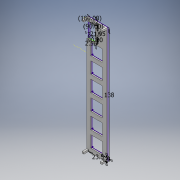
# Autodesk Inventor part: case-top
Saved by Autodesk Inventor 2017 (Build 210142000, 142)
## iProperties
Created: 2026-06-28
Part Number: case-top
Material: Generic
Document SubType Name: Modeling
Designer: hashire umamusume
Density: 1 g/cm^3
Appearance: Default
Author: hashire umamusume
Autodesk Inventor part; units mm, degrees
ref_plane "YZ Plane" through (0, 0, 0) normal (1, 0, 0) x (0, 1, 0)
ref_plane "XZ Plane" through (0, 0, 0) normal (0, 1, 0) x (-1, 0, 0)
ref_plane "XY Plane" through (0, 0, 0) normal (0, 0, 1) x (1, 0, 0)
sketch "keys" plane through (0, 0, 0) normal (0, 0, 1) x (1, 0, 0)
  line L0 (3.025, -2.525) -> (16.025, -2.525)
  line L1 (3.025, -16.525) -> (16.025, -16.525)
  line L2 (2.525, -3.025) -> (2.525, -16.025)
  line L3 (16.525, -3.025) -> (16.525, -16.025)
  arc A0 (3.025, -2.525) -> (2.525, -3.025) centre (3.025, -3.025) ccw
  arc A1 (16.525, -3.025) -> (16.025, -2.525) centre (16.025, -3.025) ccw
  arc A2 (2.525, -16.025) -> (3.025, -16.525) centre (3.025, -16.025) ccw
  arc A3 (16.025, -16.525) -> (16.525, -16.025) centre (16.025, -16.025) ccw
  line L4 (22.075, -2.525) -> (35.075, -2.525)
  line L5 (22.075, -16.525) -> (35.075, -16.525)
  line L6 (21.575, -3.025) -> (21.575, -16.025)
  line L7 (35.575, -3.025) -> (35.575, -16.025)
  arc A4 (22.075, -2.525) -> (21.575, -3.025) centre (22.075, -3.025) ccw
  arc A5 (35.575, -3.025) -> (35.075, -2.525) centre (35.075, -3.025) ccw
  arc A6 (21.575, -16.025) -> (22.075, -16.525) centre (22.075, -16.025) ccw
  arc A7 (35.075, -16.525) -> (35.575, -16.025) centre (35.075, -16.025) ccw
  line L8 (41.125, -2.525) -> (54.125, -2.525)
  line L9 (41.125, -16.525) -> (54.125, -16.525)
  line L10 (40.625, -3.025) -> (40.625, -16.025)
  line L11 (54.625, -3.025) -> (54.625, -16.025)
  arc A8 (41.125, -2.525) -> (40.625, -3.025) centre (41.125, -3.025) ccw
  arc A9 (54.625, -3.025) -> (54.125, -2.525) centre (54.125, -3.025) ccw
  arc A10 (40.625, -16.025) -> (41.125, -16.525) centre (41.125, -16.025) ccw
  arc A11 (54.125, -16.525) -> (54.625, -16.025) centre (54.125, -16.025) ccw
  line L12 (60.175, -2.525) -> (73.175, -2.525)
  line L13 (60.175, -16.525) -> (73.175, -16.525)
  line L14 (59.675, -3.025) -> (59.675, -16.025)
  line L15 (73.675, -3.025) -> (73.675, -16.025)
  arc A12 (60.175, -2.525) -> (59.675, -3.025) centre (60.175, -3.025) ccw
  arc A13 (73.675, -3.025) -> (73.175, -2.525) centre (73.175, -3.025) ccw
  arc A14 (59.675, -16.025) -> (60.175, -16.525) centre (60.175, -16.025) ccw
  arc A15 (73.175, -16.525) -> (73.675, -16.025) centre (73.175, -16.025) ccw
  line L16 (79.225, -2.525) -> (92.225, -2.525)
  line L17 (79.225, -16.525) -> (92.225, -16.525)
  line L18 (78.725, -3.025) -> (78.725, -16.025)
  line L19 (92.725, -3.025) -> (92.725, -16.025)
  arc A16 (79.225, -2.525) -> (78.725, -3.025) centre (79.225, -3.025) ccw
  arc A17 (92.725, -3.025) -> (92.225, -2.525) centre (92.225, -3.025) ccw
  arc A18 (78.725, -16.025) -> (79.225, -16.525) centre (79.225, -16.025) ccw
  arc A19 (92.225, -16.525) -> (92.725, -16.025) centre (92.225, -16.025) ccw
  line L20 (98.275, -2.525) -> (111.275, -2.525)
  line L21 (98.275, -16.525) -> (111.275, -16.525)
  line L22 (97.775, -3.025) -> (97.775, -16.025)
  line L23 (111.775, -3.025) -> (111.775, -16.025)
  arc A20 (98.275, -2.525) -> (97.775, -3.025) centre (98.275, -3.025) ccw
  arc A21 (111.775, -3.025) -> (111.275, -2.525) centre (111.275, -3.025) ccw
  arc A22 (97.775, -16.025) -> (98.275, -16.525) centre (98.275, -16.025) ccw
  arc A23 (111.275, -16.525) -> (111.775, -16.025) centre (111.275, -16.025) ccw
  point P0 (57.15, -9.525)
sketch "Sketch1" plane through (0, 0, 0) normal (0, 1, 0) x (-1, 0, 0)
  line L0 (0, 0) -> (-23.5, 0)
  line L1 (-23.5, 0) -> (-23.5, -138)
  line L2 (-23.5, -138) -> (0, -138)
  line L3 (0, -138) -> (0, 0)
  line L4 (-2, -2) -> (-21.5, -2)
  line L5 (-21.5, -2) -> (-21.5, -136)
  line L6 (-21.5, -136) -> (-2, -136)
  line L7 (-2, -136) -> (-2, -2)
  line L8 (-2, -2) -> (0, -2)
  line L9 (0, -2) -> (0, 0)
  line L10 (0, 0) -> (-2, 0)
  line L11 (-2, 0) -> (-2, -2)
  line L12 (-21.5, -2) -> (-23.5, -2)
  line L13 (-23.5, -2) -> (-23.5, 0)
  line L14 (-23.5, 0) -> (-21.5, 0)
  line L15 (-21.5, 0) -> (-21.5, -2)
  line L16 (-21.5, -136) -> (-23.5, -136)
  line L17 (-23.5, -136) -> (-23.5, -138)
  line L18 (-23.5, -138) -> (-21.5, -138)
  line L19 (-21.5, -138) -> (-21.5, -136)
  line L20 (-2, -136) -> (0, -136)
  line L21 (0, -136) -> (0, -138)
  line L22 (0, -138) -> (-2, -138)
  line L23 (-2, -138) -> (-2, -136)
  line L24 (-2, -38.4581) -> (17.5, -38.4581) construction
  line L25 (-21.5, -23.95) -> (-2, -23.95)
  line L26 (-2, -4.3088) -> (-10, -4.3088)
  line L27 (-2, -4.3088) -> (6, -4.3088) construction
  line L28 (-10, -4.3088) -> (-10, -22.3088)
  line L29 (-10, -22.3088) -> (-2, -22.3088)
  line L30 (-2, -4.3088) -> (0, -4.3088)
  line L31 (0, -4.3088) -> (0, -22.3088)
  line L32 (0, -22.3088) -> (-2, -22.3088)
  line L33 (-2, -22.3088) -> (-2, -4.3088)
  line L34 (0, -19.05) -> (0, 0)
  line L35 (-18.55, -132.7) -> (-18.55, -119.7)
  line L36 (-4.55, -132.7) -> (-4.55, -119.7)
  line L37 (-18.05, -133.2) -> (-5.05, -133.2)
  line L38 (-18.05, -119.2) -> (-5.05, -119.2)
  arc A0 (-18.55, -132.7) -> (-18.05, -133.2) centre (-18.05, -132.7) ccw
  arc A1 (-18.05, -119.2) -> (-18.55, -119.7) centre (-18.05, -119.7) ccw
  arc A2 (-5.05, -133.2) -> (-4.55, -132.7) centre (-5.05, -132.7) ccw
  arc A3 (-4.55, -119.7) -> (-5.05, -119.2) centre (-5.05, -119.7) ccw
  line L39 (-18.55, -113.65) -> (-18.55, -100.65)
  line L40 (-4.55, -113.65) -> (-4.55, -100.65)
  line L41 (-18.05, -114.15) -> (-5.05, -114.15)
  line L42 (-18.05, -100.15) -> (-5.05, -100.15)
  arc A4 (-18.55, -113.65) -> (-18.05, -114.15) centre (-18.05, -113.65) ccw
  arc A5 (-18.05, -100.15) -> (-18.55, -100.65) centre (-18.05, -100.65) ccw
  arc A6 (-5.05, -114.15) -> (-4.55, -113.65) centre (-5.05, -113.65) ccw
  arc A7 (-4.55, -100.65) -> (-5.05, -100.15) centre (-5.05, -100.65) ccw
  line L43 (-18.55, -94.6) -> (-18.55, -81.6)
  line L44 (-4.55, -94.6) -> (-4.55, -81.6)
  line L45 (-18.05, -95.1) -> (-5.05, -95.1)
  line L46 (-18.05, -81.1) -> (-5.05, -81.1)
  arc A8 (-18.55, -94.6) -> (-18.05, -95.1) centre (-18.05, -94.6) ccw
  arc A9 (-18.05, -81.1) -> (-18.55, -81.6) centre (-18.05, -81.6) ccw
  arc A10 (-5.05, -95.1) -> (-4.55, -94.6) centre (-5.05, -94.6) ccw
  arc A11 (-4.55, -81.6) -> (-5.05, -81.1) centre (-5.05, -81.6) ccw
  line L47 (-18.55, -75.55) -> (-18.55, -62.55)
  line L48 (-4.55, -75.55) -> (-4.55, -62.55)
  line L49 (-18.05, -76.05) -> (-5.05, -76.05)
  line L50 (-18.05, -62.05) -> (-5.05, -62.05)
  arc A12 (-18.55, -75.55) -> (-18.05, -76.05) centre (-18.05, -75.55) ccw
  arc A13 (-18.05, -62.05) -> (-18.55, -62.55) centre (-18.05, -62.55) ccw
  arc A14 (-5.05, -76.05) -> (-4.55, -75.55) centre (-5.05, -75.55) ccw
  arc A15 (-4.55, -62.55) -> (-5.05, -62.05) centre (-5.05, -62.55) ccw
  line L51 (-18.55, -56.5) -> (-18.55, -43.5)
  line L52 (-4.55, -56.5) -> (-4.55, -43.5)
  line L53 (-18.05, -57) -> (-5.05, -57)
  line L54 (-18.05, -43) -> (-5.05, -43)
  arc A16 (-18.55, -56.5) -> (-18.05, -57) centre (-18.05, -56.5) ccw
  arc A17 (-18.05, -43) -> (-18.55, -43.5) centre (-18.05, -43.5) ccw
  arc A18 (-5.05, -57) -> (-4.55, -56.5) centre (-5.05, -56.5) ccw
  arc A19 (-4.55, -43.5) -> (-5.05, -43) centre (-5.05, -43.5) ccw
  line L55 (-18.55, -37.45) -> (-18.55, -24.45)
  line L56 (-4.55, -37.45) -> (-4.55, -24.45)
  line L57 (-18.05, -37.95) -> (-5.05, -37.95)
  line L58 (-18.05, -23.95) -> (-5.05, -23.95)
  arc A20 (-18.55, -37.45) -> (-18.05, -37.95) centre (-18.05, -37.45) ccw
  arc A21 (-18.05, -23.95) -> (-18.55, -24.45) centre (-18.05, -24.45) ccw
  arc A22 (-5.05, -37.95) -> (-4.55, -37.45) centre (-5.05, -37.45) ccw
  arc A23 (-4.55, -24.45) -> (-5.05, -23.95) centre (-5.05, -24.45) ccw
  dimension "d0" = 23.5
  dimension "d1" = 138
  dimension "d2" = 2
  dimension "d3" = 2
  dimension "d5" = 2
  dimension "d6" = 2
  dimension "d8" = 21.95
  dimension "d24" = 8
  dimension "d25" = 180
  dimension "d26" = 18
  dimension "d27" = 90
  dimension "d28" = 90
  dimension "d31" = 0
  dimension "d32" = 2.55
  constraints: 70 end point, 14 parallel, 10 horizontal, 9 perpendicular, 7 point on line, 1 collinear
  measures "d0" distance of L2.end L1.end
  measures "d1" distance of L1.end L0.end
  measures "d2" distance between parallel lines of L2 L6
  measures "d3" distance between parallel lines of L5 L1
  measures "d5" distance between parallel lines of L0 L4
  measures "d6" distance between parallel lines of L3 L7
  measures "d8" distance between parallel lines of L4 L25
  measures "d24" distance of L26.start L26.end
  measures "d25" angle of L26 L27
  measures "d26" distance of L26.end L28.end
  measures "d27" angle of L28 L26
  measures "d28" angle of L29 L28
  measures "d31" vertical extent of L25
extrude "Extrusion1" add sketch "Sketch1" against normal blind 1.6 contours L3 L8 L11 L0 | L11 L4 L15 L0 | L3 L30 L7 L8 | L15 L12 L1 L0 | L7 L26 L28 L29 L25 L5 L4 | L3 L32 L7 L30 | L5 L16 L1 L12 | L7 L29 L28 L26 | L25 A21 L55 A20 L57 A22 L56 A23 L7 L6 L5 | L32 L3 L20 L7 | L16 L19 L2 L1 | L6 L23 L2 L19 | L25 A23 L56 A22 L57 A20 L55 A21 | L3 L2 L23 L20 | L35 A1 L38 A3 L36 A2 L37 A0 | L39 A5 L42 A7 L40 A6 L41 A4 | L43 A9 L46 A11 L44 A10 L45 A8 | L47 A13 L50 A15 L48 A14 L49 A12 | L51 A17 L54 A19 L52 A18 L53 A16
extrude "Extrusion2" add sketch "Sketch1" against normal blind 7 contours L3 L8 L11 L0 | L15 L12 L1 L0 | L16 L19 L2 L1 | L3 L2 L23 L20
extrude "Extrusion4" cut sketch "Sketch1" against normal blind 3 contours L3 L32 L7 L30 | L7 L29 L28 L26 | L25 A23 L56 A22 L57 A20 L55 A21 | L35 A1 L38 A3 L36 A2 L37 A0 | L39 A5 L42 A7 L40 A6 L41 A4 | L43 A9 L46 A11 L44 A10 L45 A8 | L47 A13 L50 A15 L48 A14 L49 A12 | L51 A17 L54 A19 L52 A18 L53 A16
body "Solid1"
